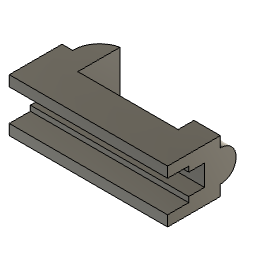
Robocon Task 1b (Autodesk Fusion 360 design; units mm, degrees)
Autodesk Fusion 360 part; units mm, degrees
note: some values were not read from the file. Set by a fixed rule: which sketch regions a step uses.
sketch "Sketch1" plane through (0, 0, 0) normal (0, 0, 1) x (1, 0, 0)
  line L0 (0, 0) -> (0, 50)
  line L1 (0, 50) -> (10, 50)
  line L2 (30, 50) -> (30, 75)
  line L3 (30, 75) -> (30, 35)
  arc A0 (30, 75) -> (10, 50) centre (35.3698, 50.2041) ccw
  line L4 (30, 35) -> (125, 35)
  line L5 (125, 35) -> (125, 50)
  line L6 (125, 50) -> (150, 50)
  line L7 (150, 50) -> (150, 0)
  line L8 (150, 0) -> (0, 0)
  constraint coincident L0.start L8.end
  constraint vertical L0
  constraint perpendicular L0 L1
  constraint perpendicular L3 L4
  constraint perpendicular L4 L5
  constraint perpendicular L5 L6
  constraint perpendicular L6 L7
  constraint perpendicular L0 L8
extrude "Extrude1" add sketch "Sketch1" along normal blind 50
sketch "Sketch2" plane through (150, 0, 0) normal (1, 0, 0) x (0, 1, 0)
  line L0 (0, 0) -> (50, 0)
  line L1 (50, 0) -> (50, 50)
  line L2 (50, 50) -> (0, 50)
  line L3 (0, 50) -> (0, 0)
  circle A0 centre (50, 25) radius 15
  constraint midpoint L1 A0.centre
extrude "Extrude2" add sketch "Sketch2" against normal blind 25 contours L1 A0 picked at (54.9491, 25.7116)
sketch "Sketch3" plane through (0, 35, 0) normal (0, 1, 0) x (-1, 0, 0)
  line L0 (-125, 0) -> (-30, 0)
  line L1 (-30, 0) -> (-30, 50)
  line L2 (-30, 50) -> (-125, 50)
  line L3 (-125, 50) -> (-125, 0)
  line L4 (-125, 15) -> (-30, 15)
  line L5 (-30, 15) -> (-30, 35)
  line L6 (-30, 35) -> (-125, 35)
  line L7 (-125, 35) -> (-125, 15)
  constraint horizontal L4
  constraint perpendicular L4 L5
  constraint parallel L4 L6
  constraint parallel L5 L7
  constraint coincident L3 L4.start
extrude "Extrude3" add sketch "Sketch3" along normal blind 10 contours L1 L3 L4 L5 L6 L7
sketch "Sketch4" plane through (0, 0, 0) normal (0, -1, 0) x (1, 0, 0)
  line L0 (0, 0) -> (150, 0)
  line L1 (150, 0) -> (150, 50)
  line L2 (150, 50) -> (0, 50)
  line L3 (0, 50) -> (0, 0)
  line L4 (0, 10) -> (150, 10)
  line L5 (150, 10) -> (150, 40)
  line L6 (150, 40) -> (0, 40)
  line L7 (0, 40) -> (0, 10)
  line L8 (150, 35) -> (0, 35)
  line L9 (0, 35) -> (0, 15)
  line L10 (0, 15) -> (150, 15)
  line L11 (150, 15) -> (150, 35)
  constraint horizontal L4
  constraint perpendicular L4 L5
  constraint parallel L4 L6
  constraint parallel L5 L7
  constraint coincident L3 L4.start
  constraint horizontal L8
  constraint perpendicular L8 L9
  constraint parallel L8 L10
  constraint parallel L9 L11
  constraint coincident L1 L8.start
  constraint coincident L5 L8.start
extrude "Extrude4" cut sketch "Sketch4" against normal blind 35 contours L1 L3 L5 L7 L8 L9 L10 L11
extrude "Extrude5" cut sketch "Sketch4" against normal blind 20 contours L1 L3 L4 L5 L7 L10 | L1 L3 L5 L6 L7 L8
